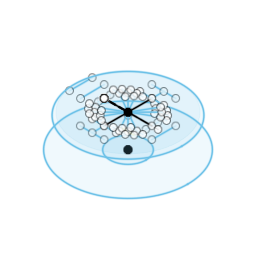
INJECTOR FILE FOR 3D PRINTING(TEST  MODEL 2) v1 (Autodesk Fusion 360 design; units mm, degrees)
Autodesk Fusion 360 part; units mm, degrees
sketch "Sketch1" plane through (0, 0, 0) normal (0, 0, 1) x (1, 0, 0)
  circle A0 centre (0, 0) radius 50
  constraint coincident A0.centre origin
extrude "Extrude1" add sketch "Sketch1" along normal blind 30
ref_plane "WorkPlane1" through (0, 0, 25) normal (0, 0, 1) x (1, 0, 0)
sketch "Sketch2" plane through (0, 0, 25) normal (0, 0, 1) x (1, 0, 0)
  circle A0 centre (0, 0) radius 45
extrude "Extrude2" cut sketch "Sketch2" along normal blind 5
sketch "Sketch3" plane through (0, 0, 0) normal (0, 0, 1) x (1, 0, 0)
  circle A0 centre (0, 0) radius 15
  constraint coincident A0.centre origin
sketch "Sketch4" plane through (0, 0, 25) normal (0, 0, 1) x (1, 0, 0)
sketch "Sketch5" plane through (0, 0, 0) normal (1, 0, 0) x (0, 1, 0)
sketch "Sketch6" plane through (0, 0, 0) normal (1, 0, 0) x (0, 1, 0)
sketch "Sketch7" plane through (0, 0, 25) normal (0, 0, 1) x (1, 0, 0)
sketch "Sketch8" plane through (0, 0, 0) normal (1, 0, 0) x (0, 1, 0)
ref_plane "WorkPlane2" through (50, 0, 0) normal (1, 0, 0) x (0, 1, 0)
sketch "Sketch9" plane through (50, 0, 0) normal (1, 0, 0) x (0, 1, 0)
extrude "Extrude3" add sketch "Sketch3" against normal blind 25
sketch "Sketch10" plane through (45, 10, 12.9326) normal (1, 0, 0) x (0, 1, 0)
ref_plane "WorkPlane4" through (51, 0, 0) normal (1, 0, 0) x (0, 1, 0)
sketch "Sketch11" plane through (51, 0, 0) normal (1, 0, 0) x (0, 1, 0)
shell "Shell1" thickness 2.286 outward yes removed faces 1 at (0.9463, -5.6032, -25)
sketch "Sketch12" plane through (0, 0, 0) normal (1, 0, 0) x (0, 1, 0)
ref_plane "WorkPlane5" through (-47, 0, 0) normal (1, 0, 0) x (0, 1, 0)
sketch "Sketch13" plane through (-47, 0, 0) normal (1, 0, 0) x (0, 1, 0)
sketch "Sketch14" plane through (0, 0, 27.286) normal (0, 0, 1) x (-1, 0, 0)
  circle A0 centre (0, 0) radius 42.714
  line L0 (0, 0) -> (-20, 0)
  line L1 (0, 0) -> (0, -20)
  line L2 (0, 0) -> (0, 20)
  line L3 (0, 0) -> (20, 0)
  line L4 (10, -20) -> (-10, -20)
  line L5 (10, 20) -> (-10, 20)
  line L6 (0, 0) -> (-25.164, 0) construction
  line L7 (0, 0) -> (20, 0) construction
  line L8 (0, 0) -> (-14.1421, -14.1421)
  line L9 (0, 0) -> (20, 0) construction
  line L10 (0, 0) -> (14.1421, -14.1421)
  line L11 (0, 0) -> (20, 0) construction
  line L12 (0, 0) -> (-14.1421, 14.1421)
  line L13 (0, 0) -> (20, 0) construction
  line L14 (0, 0) -> (14.1421, 14.1421)
  line L15 (0, 0) -> (20, 0) construction
  line L16 (0, 0) -> (10, -17.3205)
  line L17 (0, 0) -> (20, 0) construction
  line L18 (0, 0) -> (-10, -17.3205)
  line L19 (0, 0) -> (20, 0) construction
  line L20 (0, 0) -> (10, 17.3205)
  line L21 (0, 0) -> (20, 0) construction
  line L22 (0, 0) -> (-10, 17.3205)
  line L23 (0, 0) -> (20, 0) construction
  line L24 (0, 0) -> (17.3205, -10)
  line L25 (0, 0) -> (20, 0) construction
  constraint coincident A0.centre L0.start
  constraint horizontal L0
  constraint perpendicular L0 L1
  constraint perpendicular L0 L2
  constraint perpendicular L2 L3
  constraint horizontal L4
  constraint perpendicular L2 L5
  constraint horizontal L6
  constraint horizontal L7
  constraint horizontal L9
  constraint perpendicular L8 L10
  constraint horizontal L11
  constraint horizontal L13
  constraint horizontal L15
  constraint perpendicular L12 L14
  constraint horizontal L17
  constraint horizontal L19
  constraint horizontal L21
  constraint horizontal L23
  constraint horizontal L25
  constraint perpendicular L18 L24
sketch "Sketch15" plane through (0, 0, 27.286) normal (0, 0, 1) x (-1, 0, 0)
  line L0 (0, 0) -> (-17.3205, -10)
  line L1 (0, 0) -> (20, 0) construction
  line L2 (0, 0) -> (-17.3205, 10)
  line L3 (0, 0) -> (20, 0) construction
  line L4 (0, 0) -> (17.3205, 10)
  line L5 (0, 0) -> (20, 0) construction
  constraint horizontal L1
  constraint coincident L0.start L1.start
  constraint horizontal L3
  constraint horizontal L5
sketch "Sketch16" plane through (0, 0, 27.286) normal (0, 0, 1) x (-1, 0, 0)
  line L0 (20, 5) -> (20, -5)
  line L1 (-20, 5) -> (-20, -5)
  line L2 (40, 9) -> (40, -10)
  line L3 (29.754, 10) -> (30, -10)
  line L4 (-30, 10) -> (-30, -10)
  line L5 (0, 20) -> (0, 30)
  line L6 (-10, 30) -> (10, 30)
  line L7 (0, -20) -> (0, -30)
  line L8 (-10, -30) -> (10, -30)
  dimension "d102" = 10
  constraint vertical L0
  constraint vertical L1
  constraint vertical L5
  constraint horizontal L6
  constraint vertical L7
  constraint horizontal L8
  measures "d102" distance of L5.start L5.end
ref_plane "WorkPlane6" through (20, 0, 27.286) normal (-0.707107, 0, 0.707107) x (0, 1, 0)
ref_plane "WorkPlane7" through (-20, 0, 27.286) normal (0.707107, 0, 0.707107) x (0, 1, 0)
sketch "Sketch17" plane through (0, 0, 27.286) normal (0, 0, 1) x (-1, 0, 0)
sketch "Sketch18" plane through (0, 0, 27.286) normal (0, 0, 1) x (-1, 0, 0)
sketch "Sketch19" plane through (0, 0, 27.286) normal (0, 0, 1) x (-1, 0, 0)
  line L0 (15, -17.3207) -> (5, -17.3207)
  line L1 (19.142, -14.1421) -> (9.142, -14.1421)
  line L2 (22.3203, -10.0001) -> (12.3203, -10.0001)
  line L3 (19.1419, 14.1423) -> (9.1419, 14.1423)
  line L4 (14.9999, 17.3204) -> (4.9999, 17.3204)
  line L5 (-9.2177, 14.1422) -> (-19.2177, 14.1422)
  line L6 (-12.3204, 9.9999) -> (-22.3204, 9.9999)
  line L7 (22.3202, 10) -> (12.3202, 10)
  line L8 (-5.0002, 17.3207) -> (-15.0002, 17.3207)
  constraint horizontal L0
  constraint horizontal L1
  constraint horizontal L2
  constraint horizontal L4
  constraint horizontal L6
  constraint horizontal L7
  constraint horizontal L3
  constraint horizontal L8
sketch "Sketch20" plane through (0, 0, 27.286) normal (0, 0, 1) x (-1, 0, 0)
  line L0 (-5.0001, -17.3205) -> (-15.0001, -17.3205)
  line L1 (-9.1421, -14.1422) -> (-19.1421, -14.1422)
  line L2 (-12.3207, -10.0005) -> (-22.3207, -10.0005)
  constraint horizontal L2
  constraint horizontal L0
  constraint horizontal L1
hidden bodies 1
